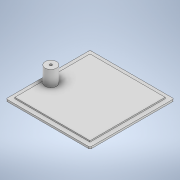
# Autodesk Inventor part: tampa caixa armazenamneto
Saved by Autodesk Inventor 2022 (Build 260153000, 153)
## iProperties
Created: 2022-03-29
Part Number: tampa caixa armazenamneto
Material: Genérico
Document SubType Name: Modeling
Designer: Hanter
Density: 1 g/cm^3
Appearance: Padrão
Author: Hanter
Autodesk Inventor part; units mm, degrees
ref_plane "YZ Plane" through (0, 0, 0) normal (1, 0, 0) x (0, 1, 0)
ref_plane "XZ Plane" through (0, 0, 0) normal (0, 1, 0) x (-1, 0, 0)
ref_plane "XY Plane" through (0, 0, 0) normal (0, 0, 1) x (1, 0, 0)
sketch "Esboço1" plane through (0, 0, 0) normal (0, 1, 0) x (-1, 0, 0)
  line L0 (-66.5, 66.5) -> (66.5, 66.5)
  line L1 (66.5, 66.5) -> (66.5, -66.5)
  line L2 (66.5, -66.5) -> (-66.5, -66.5)
  line L3 (-66.5, -66.5) -> (-66.5, 66.5)
  line L4 (-66.5, 66.5) -> (66.5, -66.5) construction
  line L5 (66.5, 66.5) -> (-66.5, -66.5) construction
  point P0 (0, 0)
  dimension "d0" = 133
  dimension "d1" = 133
  constraints: 12 end point, 2 midpoint, 2 parallel, 1 horizontal, 1 perpendicular
  measures "d0" distance of L1.end L2.end
  measures "d1" distance of L0.end L1.end
extrude "Extrusão1" add sketch "Esboço1" along normal blind 3
sketch "Esboço2" plane through (0, 3, 0) normal (0, 1, 0) x (1, 0, 0)
  line L0 (59.5, -59.5) -> (-59.5, -59.5)
  line L1 (-59.5, -59.5) -> (-59.5, 59.5)
  line L2 (-59.5, 59.5) -> (59.5, 59.5)
  line L3 (59.5, 59.5) -> (59.5, -59.5)
  line L4 (59.5, -59.5) -> (-59.5, 59.5) construction
  line L5 (-59.5, -59.5) -> (59.5, 59.5) construction
  line L6 (-66.5, 66.5) -> (-66.5, -66.5) projected
  line L7 (66.5, 66.5) -> (-66.5, 66.5) projected
  point P0 (0, 0)
  dimension "d4" = 7
  dimension "d5" = 7
  constraints: 12 end point, 2 midpoint, 2 parallel, 1 horizontal, 1 perpendicular
  measures "d4" distance between parallel lines of L6 L1
  measures "d5" distance between parallel lines of L7 L2
extrude "Extrusão2" add sketch "Esboço2" along normal blind 2
sketch "Esboço3" plane through (0, 5, 0) normal (0, 1, 0) x (1, 0, 0)
  circle A0 centre (-50.5, -11.5) radius 9
  line L0 (-66.5, -66.5) -> (66.5, -66.5) projected
  line L1 (-66.5, 66.5) -> (-66.5, -66.5) projected
  point P0 (0, 0)
  dimension "d8" = 18
  dimension "d9" = 55
  dimension "d10" = 16
  constraints: 1 centre point
  measures "d8" diameter of A0
  measures "d9" distance from line of L0 A0.centre
  measures "d10" distance from line of L1 A0.centre
extrude "Extrusão3" add sketch "Esboço3" along normal blind 25
sketch "Esboço4" plane through (0, 0, 0) normal (0, -1, 0) x (1, 0, 0)
  circle A0 centre (-50.5, 11.5) radius 9 projected
  circle A1 centre (-50.5, 11.5) radius 2
  point P0 (0, 0)
  dimension "d13" = 4
  constraints: 1 centre point, 1 coincident
  measures "d13" diameter of A1
extrude "Extrusão4" cut sketch "Esboço4" against normal blind 31.25 contours A1
sketch "Esboço5" plane through (0, 0, 0) normal (0, -1, 0) x (1, 0, 0)
  circle A0 centre (-50.5, 11.5) radius 2 projected
  circle A1 centre (-50.5, 11.5) radius 5
  point P0 (0, 0)
  dimension "d16" = 10
  constraints: 1 centre point, 1 coincident
  measures "d16" diameter of A1
extrude "Extrusão5" cut sketch "Esboço5" against normal blind 24
fillet "Arredondamento1" radius 2 4 edges at (-66.5, 1.5, -66.5) (66.5, 1.5, -66.5) (66.5, 1.5, 66.5) (-66.5, 1.5, 66.5)
